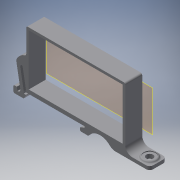
# Autodesk Inventor part: Arduino_DIN_rail_clip
Saved by Autodesk Inventor 2019.3 (Build 233278000, 278)
## iProperties
Created: 2019-03-26
Part Number: Arduino_DIN_rail_clip
Material: Generic
Document SubType Name: Modeling
Designer: erwin
Density: 1 g/cm^3
Appearance: Default
Author: erwin
Autodesk Inventor part; units mm, degrees
ref_plane "YZ Plane" through (0, 0, 0) normal (1, 0, 0) x (0, 1, 0)
ref_plane "XZ Plane" through (0, 0, 0) normal (0, 1, 0) x (-1, 0, 0)
ref_plane "XY Plane" through (0, 0, 0) normal (0, 0, 1) x (1, 0, 0)
ref_plane "Work Plane3" through (7, 2.8, -7) normal (0, 0, 1) x (1, 0, 0)
sketch "Sketch1" plane through (5.25, 2.55, -7) normal (0, 0, 1) x (1, 0, 0)
  line L0 (-4.1541, -4.2003) -> (-4.1665, -4.225)
  line L1 (-4.1665, -4.225) -> (-5.1769, -5.975)
  line L2 (-5.1769, -5.975) -> (-5.2242, -6.047)
  line L3 (-5.2242, -6.047) -> (-5.3042, -6.1384)
  line L4 (-5.3042, -6.1384) -> (-5.4132, -6.2259)
  line L5 (-5.4132, -6.2259) -> (-5.5657, -6.3032)
  line L6 (-5.5657, -6.3032) -> (-5.7236, -6.3429)
  line L7 (-5.7236, -6.3429) -> (-5.8264, -6.35)
  line L8 (-5.8264, -6.35) -> (-10.797, -6.35)
  line L9 (-10.797, -6.35) -> (-10.8813, -6.3452)
  line L10 (-10.8813, -6.3452) -> (-10.9966, -6.3229)
  line L11 (-10.9966, -6.3229) -> (-11.1155, -6.279)
  line L12 (-11.1155, -6.279) -> (-11.2275, -6.2141)
  line L13 (-11.2275, -6.2141) -> (-11.3273, -6.1303)
  line L14 (-11.3273, -6.1303) -> (-11.4111, -6.0306)
  line L15 (-11.4111, -6.0306) -> (-11.476, -5.9185)
  line L16 (-11.476, -5.9185) -> (-11.5199, -5.7996)
  line L17 (-11.5199, -5.7996) -> (-11.5422, -5.6843)
  line L18 (-11.5422, -5.6843) -> (-11.547, -5.6)
  line L19 (-11.547, -5.6) -> (-11.547, -3.1)
  line L20 (-11.547, -3.1) -> (-11.5422, -3.0157)
  line L21 (-11.5422, -3.0157) -> (-11.5199, -2.9004)
  line L22 (-11.5199, -2.9004) -> (-11.476, -2.7815)
  line L23 (-11.476, -2.7815) -> (-11.4111, -2.6694)
  line L24 (-11.4111, -2.6694) -> (-11.3273, -2.5697)
  line L25 (-11.3273, -2.5697) -> (-11.2276, -2.4859)
  line L26 (-11.2276, -2.4859) -> (-11.1155, -2.421)
  line L27 (-11.1155, -2.421) -> (-10.9966, -2.3771)
  line L28 (-10.9966, -2.3771) -> (-10.8813, -2.3548)
  line L29 (-10.8813, -2.3548) -> (-10.797, -2.35)
  line L30 (-10.797, -2.35) -> (-9.547, -2.35)
  line L31 (-9.547, -2.35) -> (-9.5261, -2.4684)
  line L32 (-9.5261, -2.4684) -> (-9.3405, -3.5211)
  line L33 (-9.3405, -3.5211) -> (-9.1943, -4.35)
  line L34 (-9.1943, -4.35) -> (-8.9511, -4.35)
  line L35 (-8.9511, -4.35) -> (-8.7503, -4.3365)
  line L36 (-8.7503, -4.3365) -> (-8.5531, -4.2963)
  line L37 (-8.5531, -4.2963) -> (-8.3631, -4.23)
  line L38 (-8.3631, -4.23) -> (-8.1837, -4.1389)
  line L39 (-8.1837, -4.1389) -> (-8.0181, -4.0245)
  line L40 (-8.0181, -4.0245) -> (-7.8693, -3.8891)
  line L41 (-7.8693, -3.8891) -> (-7.7399, -3.7349)
  line L42 (-7.7399, -3.7349) -> (-7.6324, -3.5649)
  line L43 (-7.6324, -3.5649) -> (-7.5486, -3.3819)
  line L44 (-7.5486, -3.3819) -> (-7.49, -3.1894)
  line L45 (-7.49, -3.1894) -> (-7.4577, -2.9908)
  line L46 (-7.4577, -2.9908) -> (-7.4523, -2.7896)
  line L47 (-7.4523, -2.7896) -> (-7.4739, -2.5895)
  line L48 (-7.4739, -2.5895) -> (-9.7639, 10.3976)
  line L49 (-9.7639, 10.3976) -> (-9.7977, 10.6669)
  line L50 (-9.7977, 10.6669) -> (-9.8049, 10.9381)
  line L51 (-9.8049, 10.9381) -> (-9.7853, 11.2088)
  line L52 (-9.7853, 11.2088) -> (-9.7391, 11.4762)
  line L53 (-9.7391, 11.4762) -> (-9.6668, 11.7378)
  line L54 (-9.6668, 11.7378) -> (-9.5691, 11.991)
  line L55 (53.5591, -1.7212) -> (53.53, -2.0814)
  line L56 (53.53, -2.0814) -> (53.4741, -2.4385)
  line L57 (51.58, -5.4188) -> (51.2804, -5.621)
  line L58 (51.2804, -5.621) -> (50.9666, -5.8003)
  line L59 (50.9666, -5.8003) -> (50.6403, -5.9557)
  line L60 (50.6403, -5.9557) -> (50.3033, -6.0862)
  line L61 (50.3033, -6.0862) -> (49.9575, -6.1913)
  line L62 (49.9575, -6.1913) -> (49.6049, -6.2702)
  line L63 (49.6049, -6.2702) -> (49.2473, -6.3226)
  line L64 (49.2473, -6.3226) -> (48.8868, -6.3482)
  line L65 (48.8868, -6.3482) -> (48.5254, -6.3468)
  line L66 (48.5254, -6.3468) -> (48.1651, -6.3184)
  line L67 (48.1651, -6.3184) -> (47.808, -6.2632)
  line L68 (47.808, -6.2632) -> (47.4559, -6.1816)
  line L69 (47.4559, -6.1816) -> (47.111, -6.0738)
  line L70 (47.111, -6.0738) -> (46.775, -5.9406)
  line L71 (46.775, -5.9406) -> (46.4499, -5.7828)
  line L72 (46.4499, -5.7828) -> (46.1375, -5.6011)
  line L73 (46.1375, -5.6011) -> (45.8396, -5.3965)
  line L74 (45.8396, -5.3965) -> (45.5577, -5.1703)
  line L75 (45.5577, -5.1703) -> (45.2935, -4.9238)
  line L76 (45.2935, -4.9238) -> (44.952, -4.5998)
  line L77 (44.952, -4.5998) -> (44.5921, -4.2963)
  line L78 (44.5921, -4.2963) -> (44.2151, -4.0144)
  line L79 (44.2151, -4.0144) -> (43.8222, -3.755)
  line L80 (43.8222, -3.755) -> (43.4149, -3.519)
  line L81 (43.4149, -3.519) -> (42.9944, -3.3073)
  line L82 (42.9944, -3.3073) -> (42.5623, -3.1205)
  line L83 (42.5623, -3.1205) -> (42.12, -2.9593)
  line L84 (42.12, -2.9593) -> (41.6691, -2.8242)
  line L85 (41.6691, -2.8242) -> (41.211, -2.7157)
  line L86 (41.211, -2.7157) -> (40.7473, -2.6342)
  line L87 (40.7473, -2.6342) -> (40.2797, -2.5799)
  line L88 (40.2797, -2.5799) -> (39.8097, -2.5531)
  line L89 (39.8097, -2.5531) -> (39.339, -2.5538)
  line L90 (39.339, -2.5538) -> (38.869, -2.582)
  line L91 (38.869, -2.582) -> (38.4016, -2.6377)
  line L92 (38.4016, -2.6377) -> (37.9382, -2.7205)
  line L93 (37.9382, -2.7205) -> (37.4804, -2.8304)
  line L94 (37.4804, -2.8304) -> (37.0299, -2.9668)
  line L95 (37.0299, -2.9668) -> (36.5881, -3.1293)
  line L96 (36.5881, -3.1293) -> (36.1565, -3.3174)
  line L97 (36.1565, -3.3174) -> (35.7367, -3.5303)
  line L98 (35.7367, -3.5303) -> (35.33, -3.7675)
  line L99 (35.33, -3.7675) -> (34.9379, -4.028)
  line L100 (34.9379, -4.028) -> (34.5617, -4.311)
  line L101 (34.5617, -4.311) -> (34.2028, -4.6156)
  line L102 (34.2028, -4.6156) -> (33.8622, -4.9406)
  line L103 (33.8622, -4.9406) -> (33.5412, -5.2849)
  line L104 (33.5412, -5.2849) -> (33.2409, -5.6474)
  line L105 (33.2409, -5.6474) -> (32.9623, -6.0269)
  line L106 (32.9623, -6.0269) -> (32.8779, -6.1286)
  line L107 (32.8779, -6.1286) -> (32.759, -6.2263)
  line L108 (32.759, -6.2263) -> (32.6447, -6.2884)
  line L109 (32.6447, -6.2884) -> (32.531, -6.3275)
  line L110 (32.531, -6.3275) -> (32.4233, -6.3468)
  line L111 (32.4233, -6.3468) -> (32.345, -6.3509)
  line L112 (32.345, -6.3509) -> (28.5, -6.3509)
  line L113 (28.5, -6.3509) -> (28.4157, -6.3462)
  line L114 (28.4157, -6.3462) -> (28.3004, -6.3239)
  line L115 (28.3004, -6.3239) -> (28.1815, -6.2799)
  line L116 (28.1815, -6.2799) -> (28.0694, -6.215)
  line L117 (28.0694, -6.215) -> (27.9697, -6.1313)
  line L118 (27.9697, -6.1313) -> (27.8859, -6.0315)
  line L119 (27.8859, -6.0315) -> (27.821, -5.9194)
  line L120 (27.821, -5.9194) -> (27.7771, -5.8006)
  line L121 (27.7771, -5.8006) -> (27.7548, -5.6853)
  line L122 (27.7548, -5.6853) -> (27.75, -5.6009)
  line L123 (27.75, -5.6009) -> (27.75, -4.8761)
  line L124 (27.75, -4.8761) -> (27.7548, -4.7918)
  line L125 (27.7548, -4.7918) -> (27.777, -4.6765)
  line L126 (27.777, -4.6765) -> (27.8209, -4.5577)
  line L127 (27.8209, -4.5577) -> (27.8856, -4.4459)
  line L128 (27.8856, -4.4459) -> (27.9686, -4.3469)
  line L129 (27.9686, -4.3469) -> (28.0652, -4.265)
  line L130 (28.0652, -4.265) -> (28.1659, -4.2046)
  line L131 (28.1659, -4.2046) -> (28.2435, -4.1713)
  line L132 (28.2435, -4.1713) -> (30.3355, -3.4099)
  line L133 (30.3355, -3.4099) -> (30.3544, -3.4019)
  line L134 (30.3544, -3.4019) -> (30.3653, -3.3966)
  line L135 (30.3653, -3.3966) -> (30.3801, -3.3884)
  line L136 (30.3801, -3.3884) -> (30.3958, -3.3772)
  line L137 (30.3958, -3.3772) -> (30.4081, -3.3686)
  line L138 (30.4081, -3.3686) -> (30.4268, -3.351)
  line L139 (30.4268, -3.351) -> (30.4382, -3.3394)
  line L140 (30.4382, -3.3394) -> (30.4552, -3.3168)
  line L141 (30.4552, -3.3168) -> (30.4627, -3.3063)
  line L142 (30.4627, -3.3063) -> (30.4693, -3.2938)
  line L143 (30.4693, -3.2938) -> (30.4802, -3.2723)
  line L144 (30.4802, -3.2723) -> (30.4882, -3.2496)
  line L145 (30.4882, -3.2496) -> (30.4921, -3.237)
  line L146 (30.4921, -3.237) -> (30.4979, -3.2043)
  line L147 (30.4979, -3.2043) -> (30.4988, -3.1994)
  line L148 (30.4988, -3.1994) -> (30.4989, -3.1984)
  line L149 (30.4989, -3.1984) -> (30.5, -3.1749)
  line L150 (30.5, -3.1749) -> (30.5, -2.8)
  line L151 (30.5, -2.8) -> (30.499, -2.7794)
  line L152 (30.499, -2.7794) -> (30.4977, -2.7673)
  line L153 (30.4977, -2.7673) -> (30.495, -2.7504)
  line L154 (30.495, -2.7504) -> (30.4897, -2.7315)
  line L155 (30.4897, -2.7315) -> (30.4858, -2.7169)
  line L156 (30.4858, -2.7169) -> (30.4751, -2.6926)
  line L157 (30.4751, -2.6926) -> (30.468, -2.6778)
  line L158 (30.468, -2.6778) -> (30.4511, -2.6524)
  line L159 (30.4511, -2.6524) -> (30.4439, -2.6422)
  line L160 (30.4439, -2.6422) -> (30.4353, -2.633)
  line L161 (30.4353, -2.633) -> (30.415, -2.6123)
  line L162 (30.415, -2.6123) -> (30.3999, -2.6005)
  line L163 (30.3999, -2.6005) -> (30.3824, -2.588)
  line L164 (30.3824, -2.588) -> (30.3631, -2.5774)
  line L165 (30.3631, -2.5774) -> (30.3478, -2.57)
  line L166 (30.3478, -2.57) -> (30.3232, -2.5613)
  line L167 (30.3232, -2.5613) -> (30.312, -2.5579)
  line L168 (30.312, -2.5579) -> (30.2788, -2.552)
  line L169 (30.2788, -2.552) -> (30.2743, -2.5512)
  line L170 (30.2743, -2.5512) -> (30.2734, -2.5511)
  line L171 (30.2734, -2.5511) -> (30.25, -2.55)
  line L172 (30.25, -2.55) -> (-3.9269, -2.55)
  line L173 (-3.9269, -2.55) -> (-6.0566, 9.5282)
  line L174 (-6.0566, 9.5282) -> (-6.0762, 9.6113)
  line L175 (-6.0762, 9.6113) -> (-6.1184, 9.7212)
  line L176 (-6.1184, 9.7212) -> (-6.1826, 9.8307)
  line L177 (-6.1826, 9.8307) -> (-6.2662, 9.9297)
  line L178 (-6.2662, 9.9297) -> (-6.3663, 10.0132)
  line L179 (-6.3663, 10.0132) -> (-6.4796, 10.0783)
  line L180 (-6.4796, 10.0783) -> (-6.6025, 10.1228)
  line L181 (-6.6025, 10.1228) -> (-6.7313, 10.1452)
  line L182 (-6.7313, 10.1452) -> (-6.862, 10.1449)
  line L183 (-6.862, 10.1449) -> (-6.9907, 10.122)
  line L184 (-6.9907, 10.122) -> (-7.1135, 10.077)
  line L185 (-7.1135, 10.077) -> (-7.2266, 10.0114)
  line L186 (-7.2266, 10.0114) -> (-7.3271, 9.9267)
  line L187 (-7.3271, 9.9267) -> (-7.4129, 9.8232)
  line L188 (-7.4129, 9.8232) -> (-7.4827, 9.6976)
  line L189 (-7.4827, 9.6976) -> (-7.5329, 9.533)
  line L190 (-7.5329, 9.533) -> (-7.5447, 9.3703)
  line L191 (-7.5447, 9.3703) -> (-7.5338, 9.2677)
  line L192 (-7.5338, 9.2677) -> (-5.45, -2.55)
  line L193 (-5.45, -2.55) -> (-5.45, -3.85)
  line L194 (-5.45, -3.85) -> (-4.383, -3.85)
  line L195 (-4.383, -3.85) -> (-4.3536, -3.8518)
  line L196 (-4.3536, -3.8518) -> (-4.3492, -3.8524)
  line L197 (-4.3492, -3.8524) -> (-4.3064, -3.862)
  line L198 (-4.3064, -3.862) -> (-4.3061, -3.8621)
  line L199 (-4.3061, -3.8621) -> (-4.2701, -3.8771)
  line L200 (-4.2701, -3.8771) -> (-4.2514, -3.888)
  line L201 (-4.2514, -3.888) -> (-4.2297, -3.9029)
  line L202 (-4.2297, -3.9029) -> (-4.2117, -3.9183)
  line L203 (-4.2117, -3.9183) -> (-4.195, -3.9358)
  line L204 (-4.195, -3.9358) -> (-4.1809, -3.9532)
  line L205 (-4.1809, -3.9532) -> (-4.1659, -3.9772)
  line L206 (-4.1659, -3.9772) -> (-4.1578, -3.9916)
  line L207 (-4.1578, -3.9916) -> (-4.1522, -4.0062)
  line L208 (-4.1522, -4.0062) -> (-4.1423, -4.0327)
  line L209 (-4.1423, -4.0327) -> (-4.1379, -4.0538)
  line L210 (-4.1379, -4.0538) -> (-4.1342, -4.0762)
  line L211 (-4.1342, -4.0762) -> (-4.1335, -4.0989)
  line L212 (-4.1335, -4.0989) -> (-4.1336, -4.1166)
  line L213 (-4.1336, -4.1166) -> (-4.1393, -4.1554)
  line L214 (-4.1393, -4.1554) -> (-4.1394, -4.1562)
  line L215 (-4.1394, -4.1562) -> (-4.14, -4.158)
  line L216 (-4.14, -4.158) -> (-4.1522, -4.1959)
  line L217 (-4.1522, -4.1959) -> (-4.1541, -4.2003)
  line L218 (48.8868, -6.3482) -> (68.8868, -6.3482)
  line L219 (68.8868, -6.3482) -> (68.8868, -4.3482)
  line L220 (68.8868, -4.3482) -> (58.25, -4.3482)
  line L221 (-2.25, 30) -> (52.75, 30)
  line L222 (52.75, 30) -> (52.75, 0.25)
  line L223 (52.75, 0.25) -> (-2.25, 0.25)
  line L224 (-2.25, 0.25) -> (-2.25, 30)
  line L225 (-2.75, 31.5) -> (53.25, 31.5)
  line L226 (54.25, 30.5) -> (54.25, -0.3482)
  line L227 (-3.75, 17.1842) -> (-3.75, 30.5)
  arc A0 (54.25, -0.3482) -> (58.25, -4.3482) centre (58.25, -0.3482) ccw
  arc A1 (54.25, 30.5) -> (53.25, 31.5) centre (53.25, 30.5) ccw
  arc A2 (-2.75, 31.5) -> (-3.75, 30.5) centre (-2.75, 30.5) ccw
  arc A3 (-4.451, 16.2299) -> (-9.5691, 11.991) centre (-1.8263, 7.8516) ccw
  arc A4 (-4.451, 16.2299) -> (-3.75, 17.1842) centre (-4.75, 17.1842) ccw
  point P0 (-5.25, -2.55)
  point P1 (-3.75, 16.4181)
  dimension "d1" = 2
  dimension "d2" = 1.5
  dimension "d4" = 1
  dimension "d5" = 1
  constraints: 456 end point, 11 point on circle, 8 tangent, 5 centre point, 4 parallel, 3 perpendicular, 2 horizontal, 1 equal radius, 1 point on line, 1 other
  measures "d1" distance of L219.end L218.end
  measures "d2" distance between parallel lines of L224 L227
  measures "d4" radius of A1
  measures "d5" radius of A4
extrude "Extrusion1" add sketch "Sketch1" along normal blind 10
thicken "Thicken1" operation add thickness 0.5 both sides no extend neighbours yes toward (0, -1, 0) faces at (39.6667, 2.8, -3.6667)
thicken "Thicken2" operation add thickness 0.25 both sides no extend neighbours yes toward (-1, 0, 0) faces at (3, 12.3833, -3.6667)
thicken "Thicken3" operation add thickness 0.25 both sides no extend neighbours yes toward (1, 0, 0) faces at (58, 22.4667, -3.6667)
thicken "Thicken4" operation add thickness 0.25 both sides no extend neighbours yes toward (-1, 0, 0) faces at (1.5, 24.1728, -3.6667)
thicken "Thicken5" operation add thickness 0.25 both sides no extend neighbours yes toward (1, 0, 0) faces at (59.5, 22.7673, -3.6667)
fillet "Fillet1" radius 2 2 edges at (74.1368, -2.7982, 3) (74.1368, -2.7982, -7)
sketch "Sketch2" plane through (63.75, -1.7982, 3) normal (0, 1, 0) x (1, 0, 0)
  circle A0 centre (5.3868, 5) radius 4
  line L0 (10.3868, 8) -> (10.3868, 2) projected
  line L1 (0, 10) -> (8.3868, 10) construction
  line L2 (8.3868, 0) -> (0, 0) construction
  point P0 (-63.75, 3)
  dimension "d19" = 8
  dimension "d20" = 5
  dimension "d21" = 5
  dimension "d22" = 5
  constraints: 1 centre point
  measures "d19" diameter of A0
  measures "d20" distance from line of L0 A0.centre
  measures "d21" distance from line of L1 A0.centre
  measures "d22" distance from line of L2 A0.centre
extrude "Extrusion2" add sketch "Sketch2" along normal blind 1
sketch "Sketch3" plane through (69.1368, -0.7982, -2) normal (0, 1, 0) x (1, 0, 0)
  circle A0 centre (0, 0) radius 4 construction
  point P0 (-69.1368, -2)
  constraints: 1 coincident
hole "Hole1" at (69.1368, -0.7982, -2) direction (0, -1, 0) diameter 4 end through all counterbore diameter 7 counterbore depth 0.5
fillet "Fillet2" radius 1 2 edges at (65.1368, -1.7982, -2) (65.1368, -0.7982, -2)
equation "\"d22\" = d21"
body "Solid2"
